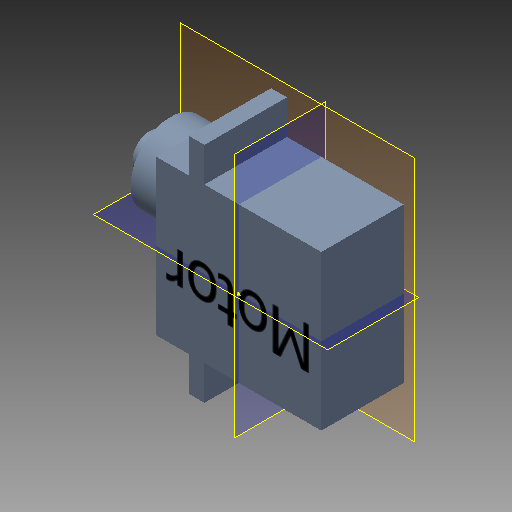
# Autodesk Inventor part: Motor Waterkanon
Saved by Autodesk Inventor 2018 (Build 220112000, 112)
## iProperties
Manager: Pierloot J.
Company: Emmaüs Bovenbouw Aalter
Created: 2015-08-18
Part Number: Motor Waterkanon
Material: S235
Catalog Web Link: http://emmausbovenbouw.op-weg.be/
Vendor: Emmaüsinstituut Bovenbouw Aalter
Document SubType Name: Modeling
Designer: Pierlootj
Engineer: Pierloot J.
Manufacturer: Standard
Standards Organization: Custom
Density: 7.86 g/cm^3
Appearance: Light Steel Blue
Title: Algemene titel
Subject: Specifieke titel
Author: Pierlootj
Keywords: Ruwe Ø xxxxx
Comments: Opmerking
Autodesk Inventor part; units mm, degrees
sketch "Sketch14" plane through (0, 0, 0) normal (0, 0, 1) x (1, 0, 0)
  line L0 (12, -11.25) -> (12, 11.25)
  line L1 (-12, 11.25) -> (-12, -11.25)
  line L2 (-12, -11.25) -> (12, 11.25) construction
  line L3 (12, -11.25) -> (-12, 11.25) construction
  line L4 (-12, 11.25) -> (5, 11.25)
  line L5 (5, 11.25) -> (5, 16.25)
  line L6 (5, 16.25) -> (7.3, 16.25)
  line L7 (7.3, 16.25) -> (7.3, 11.25)
  line L8 (5, -11.25) -> (5, -16.25)
  line L9 (5, -16.25) -> (7.3, -16.25)
  line L10 (7.3, -16.25) -> (7.3, -11.25)
  line L11 (7.3, 11.25) -> (12, 11.25)
  line L12 (7.3, -11.25) -> (12, -11.25)
  line L13 (-12, -11.25) -> (5, -11.25)
  line L14 (7.3, -11.25) -> (7.3, -16.25)
  line L15 (5, -16.25) -> (5, -11.25)
  line L16 (-12, -11.25) -> (-12, 11.25)
  line L17 (5, 11.25) -> (-12, 11.25)
  line L18 (-12, -11.25) -> (5, -11.25)
  line L19 (5, -11.25) -> (5, -16.25)
  line L20 (7.3, -11.25) -> (12, -11.25)
  line L21 (12, 11.25) -> (7.3, 11.25)
  line L22 (-12, 11.25) -> (12, 11.25)
  line L23 (12, 11.25) -> (12, -11.25)
  line L24 (12, -11.25) -> (-12, -11.25)
  line L25 (-12, -11.25) -> (-12, 11.25)
  line L26 (5, 16.25) -> (7.3, 16.25)
  line L27 (7.3, 16.25) -> (7.3, 11.25)
  line L28 (7.3, 11.25) -> (5, 11.25)
  line L29 (5, 11.25) -> (5, 16.25)
  line L30 (5, -11.25) -> (7.3, -11.25)
  line L31 (7.3, -11.25) -> (7.3, -16.25)
  line L32 (7.3, -16.25) -> (5, -16.25)
  line L33 (5, -16.25) -> (5, -11.25)
  point P0 (0, 0)
  dimension "d105" = 24
  dimension "d106" = 22.5
  dimension "d107" = 17
  dimension "d108" = 5
  dimension "d109" = 2.3
  constraints: 68 end point, 13 equal length, 7 perpendicular, 5 horizontal, 2 midpoint, 1 vertical
  measures "d105" distance of L1.start L0.end
  measures "d106" distance of L0.end L0.start
  measures "d107" distance of L1.start L4.end
  measures "d108" distance of L4.end L5.end
  measures "d109" distance of L5.end L6.end
extrude "Extrusion12" add sketch "Sketch14" along normal blind 12
sketch "Sketch15" plane through (12, -11.25, 0) normal (1, 0, 0) x (0, 0, -1)
  line L0 (0, 0) -> (0, -5) projected
  line L1 (0, -5) -> (-6, -5)
  line L2 (0, -5) -> (-12, -5) projected
  line L3 (-6, -5) -> (-6, 5.75)
  circle A0 centre (-6, 5.75) radius 5.75
  point P0 (0, 11.25)
  dimension "d112" = 10.75
  dimension "d113" = 11.5
  constraints: 4 end point, 1 centre point, 1 coincident, 1 midpoint, 1 perpendicular
  measures "d112" distance of L1.end L3.end
  measures "d113" diameter of A0
extrude "Extrusion13" add sketch "Sketch15" along normal blind 4
sketch "Sketch16" plane through (16, -5.5, 6) normal (1, 0, 0) x (0, 0, -1)
  circle A0 centre (0, 0) radius 5.75 projected
  circle A1 centre (0, 0) radius 2.5
  point P0 (6, 5.5)
  dimension "d116" = 5
  constraints: 1 centre point, 1 coincident
  measures "d116" diameter of A1
extrude "Extrusion14" add sketch "Sketch16" along normal blind 3 contours A1
sketch "Sketch18" plane through (0, 0, 12) normal (0, 0, 1) x (1, 0, 0)
  line L0 (-10.7887, 4.9339) -> (3.2892, 4.9339) construction
  line L1 (3.2892, 4.9339) -> (3.2892, -9.473) construction
  line L2 (3.2892, -9.473) -> (-10.7887, -9.473) construction
  line L3 (-10.7887, -9.473) -> (-10.7887, 4.9339) construction
  point P0 (0, 0)
  constraints: 2 other
body "Solid6"
